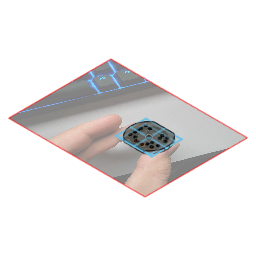
joystickFingerMount (Autodesk Fusion 360 archive; units mm, degrees)
design "joystickMount"
Autodesk Fusion 360 part; units mm, degrees
sketch "Sketch2" plane through (0, 0, 0) normal (0, 0, 1) x (1, 0, 0)
  circle A0 centre (19.3, 4.7) radius 1.0002
  circle A1 centre (23.9, 4.7) radius 1
  circle A2 centre (23.9, -1.6) radius 1
  circle A3 centre (19.3, -1.6) radius 1
  circle A4 centre (11.0258, -7.3329) radius 1
  circle A5 centre (13.6665, -7.3329) radius 1
  circle A6 centre (16.2303, -7.2816) radius 1
  circle A7 centre (4.3086, -1.2823) radius 1
  circle A8 centre (4.3086, 1.3071) radius 1
  circle A9 centre (4.3086, 3.8453) radius 1
  circle A10 centre (8.2825, -4.7434) radius 1
  circle A11 centre (8.2825, 7.5628) radius 1
  circle A12 centre (18.4095, 7.5628) radius 1
  circle A13 centre (18.4095, -4.7434) radius 1
  line L0 (2, 10) -> (26, 10)
  line L1 (26, 10) -> (26, -10)
  line L2 (26, -10) -> (2, -10)
  line L3 (2, -10) -> (2, 10)
  dimension "d1" = 2
  dimension "d2" = 2
  dimension "d3" = 2
  dimension "d4" = 2
  dimension "d5" = 2
  dimension "d6" = 2
  dimension "d7" = 2
  dimension "d8" = 2
  dimension "d9" = 2
  dimension "d10" = 2
  dimension "d11" = 2
  dimension "d12" = 2
  constraint horizontal L0
  constraint vertical L1
  constraint horizontal L2
  constraint vertical L3
  measures "d1" diameter of A1
  measures "d2" diameter of A2
  measures "d3" diameter of A4
  measures "d4" diameter of A5
  measures "d5" diameter of A6
  measures "d6" diameter of A7
  measures "d7" diameter of A8
  measures "d8" diameter of A9
  measures "d9" diameter of A10
  measures "d10" diameter of A11
  measures "d11" diameter of A12
  measures "d12" diameter of A13
extrude "Extrude1" add sketch "Sketch2" along normal blind 1
sketch "Sketch3" plane through (0, 0, 0) normal (0, 0, 1) x (1, 0, 0)
  line L0 (8.3, -8.5) -> (18.3, -8.5)
  line L1 (18.3, -8.5) -> (18.3, -4.6)
  line L2 (18.3, -4.6) -> (8.3, -4.6)
  line L3 (8.3, -4.6) -> (8.3, -8.5)
  line L4 (3.1366, 6.2847) -> (6.7858, 6.2847)
  line L5 (6.7858, 6.2847) -> (6.7858, -3.5343)
  line L6 (6.7858, -3.5343) -> (3.1366, -3.5343)
  line L7 (3.1366, -3.5343) -> (3.1366, 6.2847)
  line L8 (6.5, -5) -> (20, -5)
  line L9 (20, -5) -> (20, 9)
  line L10 (20, 9) -> (6.5, 9)
  line L11 (6.5, 9) -> (6.5, -5)
  line L12 (20, -3) -> (25.5, -3)
  line L13 (25.5, -3) -> (25.5, 6.5)
  line L14 (25.5, 6.5) -> (20, 6.5)
  line L15 (20, 6.5) -> (20, -3)
  line L16 (10.2456, 9) -> (16.0175, 9)
  line L17 (16.0175, 9) -> (16.0175, 8.206)
  line L18 (16.0175, 8.206) -> (10.2456, 8.206)
  line L19 (10.2456, 8.206) -> (10.2456, 9)
  line L20 (2, -10) -> (26, -10)
  line L21 (26, -10) -> (26, 10)
  line L22 (26, 10) -> (2, 10)
  line L23 (2, 10) -> (2, -10)
  line L24 (20, -5) -> (6.5, -5)
  line L25 (6.5, -5) -> (6.5, -6)
  line L26 (6.5, -6) -> (20, -6)
  line L27 (20, -6) -> (20, -5)
  constraint horizontal L0
  constraint vertical L1
  constraint horizontal L2
  constraint vertical L3
  constraint horizontal L4
  constraint vertical L5
  constraint horizontal L6
  constraint vertical L7
  constraint horizontal L8
  constraint vertical L9
  constraint horizontal L10
  constraint vertical L11
  constraint horizontal L12
  constraint vertical L13
  constraint horizontal L14
  constraint vertical L15
  constraint coincident L9 L12.start
  constraint horizontal L16
  constraint vertical L17
  constraint horizontal L18
  constraint vertical L19
  constraint coincident L10 L16.start
  constraint horizontal L20
  constraint vertical L21
  constraint horizontal L22
  constraint vertical L23
  constraint horizontal L24
  constraint vertical L25
  constraint horizontal L26
  constraint vertical L27
extrude "Extrude2" add sketch "Sketch3" against normal blind 1 contours L10 L16 L17 L18 L19 | L20 L21 L22 L23
sketch "Sketch4" plane through (0, 0, 0) normal (0, 0, 1) x (1, 0, 0)
  circle A0 centre (13.3, 1.5) radius 0.7133
  line L0 (13.3, 1.5) -> (28.3, 1.5)
  line L1 (28.3, 1.5) -> (28.3, 14)
  line L2 (28.3, 14) -> (13.3, 14)
  line L3 (13.3, 14) -> (13.3, 1.5)
  line L4 (13.3, 1.5) -> (28.3, 1.5)
  line L5 (28.3, 1.5) -> (28.3, -11)
  line L6 (28.3, -11) -> (13.3, -11)
  line L7 (13.3, -11) -> (13.3, 1.5)
  line L8 (13.3, 1.5) -> (-1.7, 1.5)
  line L9 (-1.7, 1.5) -> (-1.7, 14)
  line L10 (-1.7, 14) -> (13.3, 14)
  line L11 (13.3, 14) -> (13.3, 1.5)
  line L12 (13.3, 1.5) -> (-1.7, 1.5)
  line L13 (-1.7, 1.5) -> (-1.7, -11)
  line L14 (-1.7, -11) -> (13.3, -11)
  line L15 (13.3, -11) -> (13.3, 1.5)
  line L16 (26, 10) -> (2, 10)
  line L17 (2, 10) -> (2, -10)
  line L18 (2, -10) -> (26, -10)
  line L19 (26, -10) -> (26, 10)
  dimension "d19" = 15
  dimension "d20" = 12.5
  dimension "d21" = 15
  dimension "d22" = 12.5
  dimension "d23" = 15
  dimension "d24" = 12.5
  dimension "d25" = 15
  dimension "d26" = 12.5
  constraint horizontal L0
  constraint vertical L1
  constraint horizontal L2
  constraint vertical L3
  constraint coincident A0.centre L0.start
  constraint horizontal L4
  constraint vertical L5
  constraint horizontal L6
  constraint vertical L7
  constraint horizontal L8
  constraint vertical L9
  constraint horizontal L10
  constraint vertical L11
  constraint horizontal L12
  constraint vertical L13
  constraint horizontal L14
  constraint vertical L15
  constraint horizontal L16
  constraint vertical L17
  constraint horizontal L18
  constraint vertical L19
  measures "d19" distance of A0.centre L0.end
  measures "d20" distance of A0.centre L2.end
  measures "d21" distance of A0.centre L0.end
  measures "d22" distance of A0.centre L6.end
  measures "d23" distance of A0.centre L8.end
  measures "d24" distance of A0.centre L2.end
  measures "d25" distance of A0.centre L8.end
  measures "d26" distance of A0.centre L6.end
extrude "Extrude3" add sketch "Sketch4" along normal blind 1 contours L0 L1 L2 L3 L4 L11 L16 L19 | L0 L4 L5 L6 L7 L15 L18 L19 | L3 L8 L9 L10 L11 L12 L16 L17 | L7 L8 L12 L13 L14 L15 L17 L18
extrude "Extrude4" add 1 faces at (9.5333, 12.6667, 0) along direction (0, 0, -1) blind 1
sketch "Sketch5" plane through (0, 0, -1) normal (0, 0, -1) x (1, 0, 0)
  line L0 (-1.7, 11) -> (-1.7, -14)
  line L1 (-1.7, -14) -> (28.3, -14)
  line L2 (28.3, -14) -> (28.3, 11)
  line L3 (28.3, 11) -> (-1.7, 11)
  line L4 (6.5, 3.5343) -> (6.5, 6)
  line L5 (6.5, 6) -> (8.3, 6)
  line L6 (8.3, 6) -> (8.3, 8.5)
  line L7 (8.3, 8.5) -> (18.3, 8.5)
  line L8 (18.3, 8.5) -> (18.3, 6)
  line L9 (18.3, 6) -> (20, 6)
  line L10 (20, 6) -> (20, 3)
  line L11 (20, 3) -> (25.5, 3)
  line L12 (25.5, 3) -> (25.5, -6.5)
  line L13 (25.5, -6.5) -> (20, -6.5)
  line L14 (20, -6.5) -> (20, -9)
  line L15 (20, -9) -> (16.0175, -9)
  line L16 (16.0175, -9) -> (16.0175, -8.206)
  line L17 (16.0175, -8.206) -> (10.2456, -8.206)
  line L18 (10.2456, -8.206) -> (10.2456, -9)
  line L19 (10.2456, -9) -> (6.5, -9)
  line L20 (6.5, -9) -> (6.5, -6.2847)
  line L21 (6.5, -6.2847) -> (3.1366, -6.2847)
  line L22 (3.1366, -6.2847) -> (3.1366, 3.5343)
  line L23 (3.1366, 3.5343) -> (6.5, 3.5343)
  line L24 (28.3, -14) -> (22.3, -14)
  line L25 (22.3, -14) -> (22.3, -8)
  line L26 (22.3, -8) -> (28.3, -8)
  line L27 (28.3, -8) -> (28.3, -14)
  circle A0 centre (22.3, -8) radius 1
  line L28 (28.3, 11) -> (22.3, 11)
  line L29 (22.3, 11) -> (22.3, 5)
  line L30 (22.3, 5) -> (28.3, 5)
  line L31 (28.3, 5) -> (28.3, 11)
  circle A1 centre (22.3, 5) radius 1
  line L32 (-1.7, -14) -> (4.3, -14)
  line L33 (4.3, -14) -> (4.3, -8)
  line L34 (4.3, -8) -> (-1.7, -8)
  line L35 (-1.7, -8) -> (-1.7, -14)
  circle A2 centre (4.3, -8) radius 1
  line L36 (-1.7, 11) -> (4.3, 11)
  line L37 (4.3, 11) -> (4.3, 5)
  line L38 (4.3, 5) -> (-1.7, 5)
  line L39 (-1.7, 5) -> (-1.7, 11)
  circle A3 centre (4.3, 5) radius 1
  dimension "d31" = 2
  dimension "d32" = 2
  dimension "d33" = 6
  dimension "d34" = 6
  dimension "d35" = 2
  dimension "d36" = 6
  dimension "d37" = 2
  dimension "d40" = 6
  dimension "d43" = 6
  dimension "d44" = 6
  dimension "d45" = 6
  dimension "d46" = 6
  constraint horizontal L24
  constraint vertical L25
  constraint horizontal L26
  constraint vertical L27
  constraint coincident L1.end L2.start
  constraint coincident L25.end L26.start
  constraint horizontal L28
  constraint vertical L29
  constraint horizontal L30
  constraint vertical L31
  constraint coincident L2.end L3.start
  constraint coincident L29.end L30.start
  constraint horizontal L32
  constraint vertical L33
  constraint horizontal L34
  constraint vertical L35
  constraint coincident L0.end L1.start
  constraint coincident L33.end L34.start
  constraint horizontal L36
  constraint vertical L37
  constraint horizontal L38
  constraint vertical L39
  constraint coincident L0.start L3.end
  constraint coincident L37.end L38.start
  measures "d31" diameter of A0
  measures "d32" diameter of A1
  measures "d33" distance of L0.end L32.end
  measures "d34" distance of L1.end L24.end
  measures "d35" diameter of A2
  measures "d36" distance of L0.start L36.end
  measures "d37" diameter of A3
  measures "d40" distance of L1.end L26.end
  measures "d43" distance of L2.end L30.end
  measures "d44" distance of L2.end L28.end
  measures "d45" distance of L0.start L38.end
  measures "d46" distance of L0.end L34.end
extrude "Extrude5" cut sketch "Sketch5" against normal blind 2 contours L37 L38 A3 | L37 L38 A3 | L33 L34 A2 | L33 L34 A2 | L29 L30 A1 | L29 L30 A1 | L25 L26 A0 | L25 L26 A0
sketch "Sketch6" plane through (0, 0, -1) normal (0, 0, -1) x (1, 0, 0)
  circle A0 centre (4.3, 5) radius 1
  circle A1 centre (22.3, -8) radius 1
  circle A2 centre (4.3, -8) radius 1
  circle A3 centre (22.3, 5) radius 1
  line L0 (-1.7, 11) -> (-1.7, -14)
  line L1 (-1.7, -14) -> (28.3, -14)
  line L2 (28.3, -14) -> (28.3, 11)
  line L3 (28.3, 11) -> (-1.7, 11)
  line L4 (6.5, 3.5343) -> (6.5, 6)
  line L5 (6.5, 6) -> (8.3, 6)
  line L6 (8.3, 6) -> (8.3, 8.5)
  line L7 (8.3, 8.5) -> (18.3, 8.5)
  line L8 (18.3, 8.5) -> (18.3, 6)
  line L9 (18.3, 6) -> (20, 6)
  line L10 (20, 6) -> (20, 3)
  line L11 (20, 3) -> (25.5, 3)
  line L12 (25.5, 3) -> (25.5, -6.5)
  line L13 (25.5, -6.5) -> (20, -6.5)
  line L14 (20, -6.5) -> (20, -9)
  line L15 (20, -9) -> (16.0175, -9)
  line L16 (16.0175, -9) -> (16.0175, -8.206)
  line L17 (16.0175, -8.206) -> (10.2456, -8.206)
  line L18 (10.2456, -8.206) -> (10.2456, -9)
  line L19 (10.2456, -9) -> (6.5, -9)
  line L20 (6.5, -9) -> (6.5, -6.2847)
  line L21 (6.5, -6.2847) -> (3.1366, -6.2847)
  line L22 (3.1366, -6.2847) -> (3.1366, 3.5343)
  line L23 (3.1366, 3.5343) -> (6.5, 3.5343)
  circle A4 centre (13.3696, -1.5612) radius 15.0697
extrude "Extrude6" cut sketch "Sketch6" against normal blind 2 contours L0 L3 A4 | L0 L1 A4 | L2 L3 A4 | L1 L2 A4
equation "d33 = distanceFromRightLeft"
equation "d34 = distanceFromRightLeft"
equation "d36 = distanceFromRightLeft"
equation "d40 = distanceFromTopDown"
equation "distanceFromRightLeft = 6 mm"
equation "distanceFromTopDown = 6 mm"
equation "d43 = distanceFromTopDown"
equation "d44 = distanceFromRightLeft"
equation "d45 = distanceFromTopDown"
equation "d46 = distanceFromTopDown"
